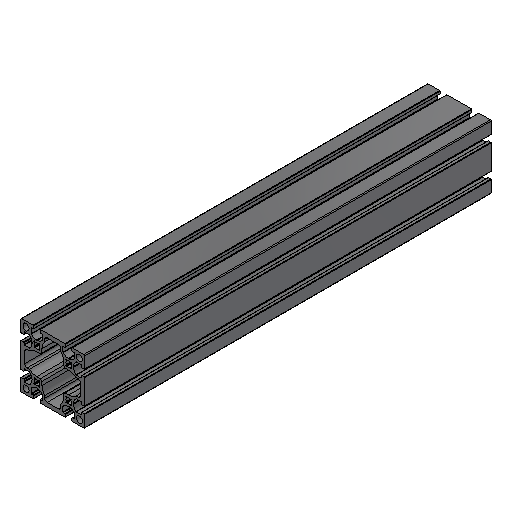
# Autodesk Inventor part: PROFILE
Saved by Autodesk Inventor 2022.5 (Build 265521000, 521)
## iProperties
Created: 2022-06-15
Part Number: PROFILE
Material: AL6061
Document SubType Name: Modeling
Designer: 박성규
Density: 2.71 g/cm^3
Description: 3
MAKER: DY PROFILE
Detail Description: Purchased products
Author: 오동하
Revision Number: A
Title: DP8080-510L
Autodesk Inventor part; units mm, degrees
ref_plane "YZ Plane" through (0, 0, 0) normal (1, 0, 0) x (0, 1, 0)
ref_plane "XZ Plane" through (0, 0, 0) normal (0, 1, 0) x (-1, 0, 0)
ref_plane "XY Plane" through (0, 0, 0) normal (0, 0, 1) x (1, 0, 0)
sketch "스케치3" plane through (0, 0, 0) normal (0, 0, 1) x (1, 0, 0)
  line L0 (20, -40) -> (20, -6.357)
  arc A0 (22.8645, -21.8316) -> (22.906, -22.2062) centre (23.1172, -21.9932) ccw
  circle A1 centre (33.5, -33.5) radius 4
  line L1 (-20, -40) -> (-20, -6.0705)
  arc A2 (22.8645, -21.8316) -> (22.8645, -18.1684) centre (20, -20) ccw
  circle A3 centre (-33.5, -33.5) radius 4
  line L2 (0, -45.1572) -> (0, 0)
  arc A4 (40, 15.3564) -> (39.5, 15.8564) centre (39.5, 15.3564) ccw
  line L3 (39.5, 15.8564) -> (36.5, 15.8564)
  arc A5 (36.5, 15.8564) -> (36, 15.3564) centre (36.5, 15.3564) ccw
  line L4 (36, 15.3564) -> (36, 13.3524)
  arc A6 (35.5, 12.8524) -> (36, 13.3524) centre (35.5, 13.3524) ccw
  line L5 (35.5, 12.8524) -> (29.4329, 12.8524)
  arc A7 (29.0959, 12.9831) -> (29.4329, 12.8524) centre (29.4329, 13.3524) ccw
  arc A8 (26.0139, 19.4861) -> (29.0959, 12.9831) centre (35.5, 20) ccw
  line L6 (26.0139, 19.4861) -> (25.5, 20)
  line L7 (25.5, 20) -> (26.0139, 20.5139)
  arc A9 (29.0959, 27.0169) -> (26.0139, 20.5139) centre (35.5, 20) ccw
  arc A10 (29.4329, 27.1476) -> (29.0959, 27.0169) centre (29.4329, 26.6476) ccw
  line L8 (29.4329, 27.1476) -> (35.5, 27.1476)
  arc A11 (36, 26.6476) -> (35.5, 27.1476) centre (35.5, 26.6476) ccw
  line L9 (36, 26.6476) -> (36, 24.6436)
  arc A12 (36, 24.6436) -> (36.5, 24.1436) centre (36.5, 24.6436) ccw
  line L10 (36.5, 24.1436) -> (39.5, 24.1436)
  arc A13 (39.5, 24.1436) -> (40, 24.6436) centre (39.5, 24.6436) ccw
  line L11 (40, 24.6436) -> (40, 38)
  line L12 (40, 38) -> (40, 39)
  arc A14 (40, 39) -> (39, 40) centre (39, 39) ccw
  line L13 (39, 40) -> (38, 40)
  line L14 (38, 40) -> (24.6436, 40)
  arc A15 (24.6436, 40) -> (24.1436, 39.5) centre (24.6436, 39.5) ccw
  line L15 (24.1436, 39.5) -> (24.1436, 36.5)
  arc A16 (24.1436, 36.5) -> (24.6436, 36) centre (24.6436, 36.5) ccw
  line L16 (24.6436, 36) -> (26.6476, 36)
  arc A17 (27.1476, 35.5) -> (26.6476, 36) centre (26.6476, 35.5) ccw
  line L17 (27.1476, 35.5) -> (27.1476, 29.4329)
  arc A18 (27.0169, 29.0959) -> (27.1476, 29.4329) centre (26.6476, 29.4329) ccw
  arc A19 (20.5139, 26.0139) -> (27.0169, 29.0959) centre (20, 35.5) ccw
  line L18 (20.5139, 26.0139) -> (20, 25.5)
  line L19 (20, 25.5) -> (19.4861, 26.0139)
  arc A20 (12.9831, 29.0959) -> (19.4861, 26.0139) centre (20, 35.5) ccw
  arc A21 (12.8524, 29.4329) -> (12.9831, 29.0959) centre (13.3524, 29.4329) ccw
  line L20 (12.8524, 29.4329) -> (12.8524, 35.5)
  arc A22 (13.3524, 36) -> (12.8524, 35.5) centre (13.3524, 35.5) ccw
  line L21 (13.3524, 36) -> (15.3564, 36)
  arc A23 (15.3564, 36) -> (15.8564, 36.5) centre (15.3564, 36.5) ccw
  line L22 (15.8564, 36.5) -> (15.8564, 39.5)
  arc A24 (15.8564, 39.5) -> (15.3564, 40) centre (15.3564, 39.5) ccw
  line L23 (15.3564, 40) -> (0, 40)
  line L24 (0, 40) -> (-15.3564, 40)
  arc A25 (-15.3564, 40) -> (-15.8564, 39.5) centre (-15.3564, 39.5) ccw
  line L25 (-15.8564, 39.5) -> (-15.8564, 36.5)
  arc A26 (-15.8564, 36.5) -> (-15.3564, 36) centre (-15.3564, 36.5) ccw
  line L26 (-15.3564, 36) -> (-13.3524, 36)
  arc A27 (-12.8524, 35.5) -> (-13.3524, 36) centre (-13.3524, 35.5) ccw
  line L27 (-12.8524, 35.5) -> (-12.8524, 29.4329)
  arc A28 (-12.9831, 29.0959) -> (-12.8524, 29.4329) centre (-13.3524, 29.4329) ccw
  arc A29 (-19.4861, 26.0139) -> (-12.9831, 29.0959) centre (-20, 35.5) ccw
  line L28 (-19.4861, 26.0139) -> (-20, 25.5)
  line L29 (-20, 25.5) -> (-20.5139, 26.0139)
  arc A30 (-27.0169, 29.0959) -> (-20.5139, 26.0139) centre (-20, 35.5) ccw
  arc A31 (-27.1476, 29.4329) -> (-27.0169, 29.0959) centre (-26.6476, 29.4329) ccw
  line L30 (-27.1476, 29.4329) -> (-27.1476, 35.5)
  arc A32 (-26.6476, 36) -> (-27.1476, 35.5) centre (-26.6476, 35.5) ccw
  line L31 (-26.6476, 36) -> (-24.6436, 36)
  arc A33 (-24.6436, 36) -> (-24.1436, 36.5) centre (-24.6436, 36.5) ccw
  line L32 (-24.1436, 36.5) -> (-24.1436, 39.5)
  arc A34 (-24.1436, 39.5) -> (-24.6436, 40) centre (-24.6436, 39.5) ccw
  line L33 (-24.6436, 40) -> (-38, 40)
  line L34 (-38, 40) -> (-39, 40)
  arc A35 (-39, 40) -> (-40, 39) centre (-39, 39) ccw
  line L35 (-40, 39) -> (-40, 38)
  line L36 (-40, 38) -> (-40, 24.6436)
  arc A36 (-40, 24.6436) -> (-39.5, 24.1436) centre (-39.5, 24.6436) ccw
  line L37 (-39.5, 24.1436) -> (-36.5, 24.1436)
  arc A37 (-36.5, 24.1436) -> (-36, 24.6436) centre (-36.5, 24.6436) ccw
  line L38 (-36, 24.6436) -> (-36, 26.6476)
  arc A38 (-35.5, 27.1476) -> (-36, 26.6476) centre (-35.5, 26.6476) ccw
  line L39 (-35.5, 27.1476) -> (-29.4329, 27.1476)
  arc A39 (-29.0959, 27.0169) -> (-29.4329, 27.1476) centre (-29.4329, 26.6476) ccw
  arc A40 (-26.0139, 20.5139) -> (-29.0959, 27.0169) centre (-35.5, 20) ccw
  line L40 (-26.0139, 20.5139) -> (-25.5, 20)
  line L41 (-25.5, 20) -> (-26.0139, 19.4861)
  arc A41 (-29.0959, 12.9831) -> (-26.0139, 19.4861) centre (-35.5, 20) ccw
  arc A42 (-29.4329, 12.8524) -> (-29.0959, 12.9831) centre (-29.4329, 13.3524) ccw
  line L42 (-29.4329, 12.8524) -> (-35.5, 12.8524)
  arc A43 (-36, 13.3524) -> (-35.5, 12.8524) centre (-35.5, 13.3524) ccw
  line L43 (-36, 13.3524) -> (-36, 15.3564)
  arc A44 (-36, 15.3564) -> (-36.5, 15.8564) centre (-36.5, 15.3564) ccw
  line L44 (-36.5, 15.8564) -> (-39.5, 15.8564)
  arc A45 (-39.5, 15.8564) -> (-40, 15.3564) centre (-39.5, 15.3564) ccw
  line L45 (-40, 15.3564) -> (-40, 0)
  line L46 (-40, 0) -> (-40, -15.3564)
  arc A46 (-40, -15.3564) -> (-39.5, -15.8564) centre (-39.5, -15.3564) ccw
  line L47 (-39.5, -15.8564) -> (-36.5, -15.8564)
  arc A47 (-36.5, -15.8564) -> (-36, -15.3564) centre (-36.5, -15.3564) ccw
  line L48 (-36, -15.3564) -> (-36, -13.3524)
  arc A48 (-35.5, -12.8524) -> (-36, -13.3524) centre (-35.5, -13.3524) ccw
  line L49 (-35.5, -12.8524) -> (-29.4329, -12.8524)
  arc A49 (-29.0959, -12.9831) -> (-29.4329, -12.8524) centre (-29.4329, -13.3524) ccw
  arc A50 (-26.0139, -19.4861) -> (-29.0959, -12.9831) centre (-35.5, -20) ccw
  line L50 (-26.0139, -19.4861) -> (-25.5, -20)
  line L51 (-25.5, -20) -> (-26.0139, -20.5139)
  arc A51 (-29.0959, -27.0169) -> (-26.0139, -20.5139) centre (-35.5, -20) ccw
  arc A52 (-29.4329, -27.1476) -> (-29.0959, -27.0169) centre (-29.4329, -26.6476) ccw
  line L52 (-29.4329, -27.1476) -> (-35.5, -27.1476)
  arc A53 (-36, -26.6476) -> (-35.5, -27.1476) centre (-35.5, -26.6476) ccw
  line L53 (-36, -26.6476) -> (-36, -24.6436)
  arc A54 (-36, -24.6436) -> (-36.5, -24.1436) centre (-36.5, -24.6436) ccw
  line L54 (-36.5, -24.1436) -> (-39.5, -24.1436)
  arc A55 (-39.5, -24.1436) -> (-40, -24.6436) centre (-39.5, -24.6436) ccw
  line L55 (-40, -24.6436) -> (-40, -38)
  line L56 (-40, -38) -> (-40, -39)
  arc A56 (-40, -39) -> (-39, -40) centre (-39, -39) ccw
  line L57 (-39, -40) -> (-38, -40)
  line L58 (-38, -40) -> (-24.6436, -40)
  arc A57 (-24.6436, -40) -> (-24.1436, -39.5) centre (-24.6436, -39.5) ccw
  line L59 (-24.1436, -39.5) -> (-24.1436, -36.5)
  arc A58 (-24.1436, -36.5) -> (-24.6436, -36) centre (-24.6436, -36.5) ccw
  line L60 (-24.6436, -36) -> (-26.6476, -36)
  arc A59 (-27.1476, -35.5) -> (-26.6476, -36) centre (-26.6476, -35.5) ccw
  line L61 (-27.1476, -35.5) -> (-27.1476, -29.4329)
  arc A60 (-27.0169, -29.0959) -> (-27.1476, -29.4329) centre (-26.6476, -29.4329) ccw
  arc A61 (-20.5139, -26.0139) -> (-27.0169, -29.0959) centre (-20, -35.5) ccw
  line L62 (-20.5139, -26.0139) -> (-20, -25.5)
  line L63 (-20, -25.5) -> (-19.4861, -26.0139)
  arc A62 (-12.9831, -29.0959) -> (-19.4861, -26.0139) centre (-20, -35.5) ccw
  arc A63 (-12.8524, -29.4329) -> (-12.9831, -29.0959) centre (-13.3524, -29.4329) ccw
  line L64 (-12.8524, -29.4329) -> (-12.8524, -35.5)
  arc A64 (-13.3524, -36) -> (-12.8524, -35.5) centre (-13.3524, -35.5) ccw
  line L65 (-13.3524, -36) -> (-15.3564, -36)
  arc A65 (-15.3564, -36) -> (-15.8564, -36.5) centre (-15.3564, -36.5) ccw
  line L66 (-15.8564, -36.5) -> (-15.8564, -39.5)
  arc A66 (-15.8564, -39.5) -> (-15.3564, -40) centre (-15.3564, -39.5) ccw
  line L67 (-15.3564, -40) -> (0, -40)
  line L68 (0, -40) -> (15.3564, -40)
  arc A67 (15.3564, -40) -> (15.8564, -39.5) centre (15.3564, -39.5) ccw
  line L69 (15.8564, -39.5) -> (15.8564, -36.5)
  arc A68 (15.8564, -36.5) -> (15.3564, -36) centre (15.3564, -36.5) ccw
  line L70 (15.3564, -36) -> (13.3524, -36)
  arc A69 (12.8524, -35.5) -> (13.3524, -36) centre (13.3524, -35.5) ccw
  line L71 (12.8524, -35.5) -> (12.8524, -29.4329)
  arc A70 (12.9831, -29.0959) -> (12.8524, -29.4329) centre (13.3524, -29.4329) ccw
  arc A71 (19.4861, -26.0139) -> (12.9831, -29.0959) centre (20, -35.5) ccw
  line L72 (19.4861, -26.0139) -> (20, -25.5)
  line L73 (20, -25.5) -> (20.5139, -26.0139)
  arc A72 (27.0169, -29.0959) -> (20.5139, -26.0139) centre (20, -35.5) ccw
  arc A73 (27.1476, -29.4329) -> (27.0169, -29.0959) centre (26.6476, -29.4329) ccw
  line L74 (27.1476, -29.4329) -> (27.1476, -35.5)
  arc A74 (26.6476, -36) -> (27.1476, -35.5) centre (26.6476, -35.5) ccw
  line L75 (26.6476, -36) -> (24.6436, -36)
  arc A75 (24.6436, -36) -> (24.1436, -36.5) centre (24.6436, -36.5) ccw
  line L76 (24.1436, -36.5) -> (24.1436, -39.5)
  arc A76 (24.1436, -39.5) -> (24.6436, -40) centre (24.6436, -39.5) ccw
  line L77 (24.6436, -40) -> (38, -40)
  line L78 (38, -40) -> (39, -40)
  arc A77 (39, -40) -> (40, -39) centre (39, -39) ccw
  line L79 (40, -39) -> (40, -38)
  line L80 (40, -38) -> (40, -24.6436)
  arc A78 (40, -24.6436) -> (39.5, -24.1436) centre (39.5, -24.6436) ccw
  line L81 (39.5, -24.1436) -> (36.5, -24.1436)
  arc A79 (36.5, -24.1436) -> (36, -24.6436) centre (36.5, -24.6436) ccw
  line L82 (36, -24.6436) -> (36, -26.6476)
  arc A80 (35.5, -27.1476) -> (36, -26.6476) centre (35.5, -26.6476) ccw
  line L83 (35.5, -27.1476) -> (29.4329, -27.1476)
  arc A81 (29.0959, -27.0169) -> (29.4329, -27.1476) centre (29.4329, -26.6476) ccw
  arc A82 (26.0139, -20.5139) -> (29.0959, -27.0169) centre (35.5, -20) ccw
  line L84 (26.0139, -20.5139) -> (25.5, -20)
  line L85 (25.5, -20) -> (26.0139, -19.4861)
  arc A83 (29.0959, -12.9831) -> (26.0139, -19.4861) centre (35.5, -20) ccw
  arc A84 (29.4329, -12.8524) -> (29.0959, -12.9831) centre (29.4329, -13.3524) ccw
  line L86 (29.4329, -12.8524) -> (35.5, -12.8524)
  arc A85 (36, -13.3524) -> (35.5, -12.8524) centre (35.5, -13.3524) ccw
  line L87 (36, -13.3524) -> (36, -15.3564)
  arc A86 (36, -15.3564) -> (36.5, -15.8564) centre (36.5, -15.3564) ccw
  line L88 (36.5, -15.8564) -> (39.5, -15.8564)
  arc A87 (39.5, -15.8564) -> (40, -15.3564) centre (39.5, -15.3564) ccw
  line L89 (40, -15.3564) -> (40, 0)
  line L90 (40, 0) -> (40, 15.3564)
  arc A88 (22.906, -17.7938) -> (22.8645, -18.1684) centre (23.1172, -18.0068) ccw
  line L91 (22.906, -17.7938) -> (23.6045, -17.1009)
  arc A89 (35, 7) -> (32, 10) centre (32, 7) ccw
  line L92 (32, 10) -> (29.0692, 10)
  arc A90 (29.0692, 10) -> (20, 13.5) centre (20, 0) ccw
  line L93 (20, 13.5) -> (15.4691, 13.5)
  line L94 (15.4691, 13.5) -> (13.5, 15.4691)
  line L95 (13.5, 15.4691) -> (13.5, 20)
  arc A91 (13.5, 20) -> (10, 29.0692) centre (0, 20) ccw
  line L96 (10, 29.0692) -> (10, 32)
  arc A92 (10, 32) -> (7, 35) centre (7, 32) ccw
  line L97 (7, 35) -> (0, 35)
  line L98 (0, 35) -> (-7, 35)
  arc A93 (-7, 35) -> (-10, 32) centre (-7, 32) ccw
  line L99 (-10, 32) -> (-10, 29.0692)
  arc A94 (-10, 29.0692) -> (-13.5, 20) centre (0, 20) ccw
  line L100 (-13.5, 20) -> (-13.5, 15.4691)
  line L101 (-13.5, 15.4691) -> (-15.4691, 13.5)
  line L102 (-15.4691, 13.5) -> (-20, 13.5)
  arc A95 (-20, 13.5) -> (-29.0692, 10) centre (-20, 0) ccw
  line L103 (-29.0692, 10) -> (-32, 10)
  arc A96 (-32, 10) -> (-35, 7) centre (-32, 7) ccw
  line L104 (-35, 7) -> (-35, 0)
  line L105 (-35, 0) -> (-35, -7)
  arc A97 (-35, -7) -> (-32, -10) centre (-32, -7) ccw
  line L106 (-32, -10) -> (-29.0692, -10)
  arc A98 (-29.0692, -10) -> (-20, -13.5) centre (-20, 0) ccw
  line L107 (-20, -13.5) -> (-15.4691, -13.5)
  line L108 (-15.4691, -13.5) -> (-13.5, -15.4691)
  line L109 (-13.5, -15.4691) -> (-13.5, -20)
  arc A99 (-13.5, -20) -> (-10, -29.0692) centre (0, -20) ccw
  line L110 (-10, -29.0692) -> (-10, -32)
  arc A100 (-10, -32) -> (-7, -35) centre (-7, -32) ccw
  line L111 (-7, -35) -> (0, -35)
  line L112 (0, -35) -> (7, -35)
  arc A101 (7, -35) -> (10, -32) centre (7, -32) ccw
  line L113 (10, -32) -> (10, -29.0692)
  arc A102 (10, -29.0692) -> (13.5, -20) centre (0, -20) ccw
  line L114 (13.5, -20) -> (13.5, -15.4691)
  line L115 (13.5, -15.4691) -> (15.4691, -13.5)
  line L116 (15.4691, -13.5) -> (20, -13.5)
  arc A103 (20, -13.5) -> (29.0692, -10) centre (20, 0) ccw
  line L117 (29.0692, -10) -> (32, -10)
  arc A104 (32, -10) -> (35, -7) centre (32, -7) ccw
  line L118 (35, -7) -> (35, 0)
  line L119 (35, 0) -> (35, 7)
  circle A105 centre (-33.5, 33.5) radius 4
  line L120 (0, 45.1572) -> (0, 0)
  line L121 (0, 0) -> (-45.8762, 0)
  line L122 (-20, 40) -> (-20, 5.3913)
  arc A106 (-17.094, 22.2062) -> (-17.1355, 21.8316) centre (-16.8828, 21.9932) ccw
  line L123 (-17.094, 22.2062) -> (-16.3955, 22.8991)
  arc A107 (-16.3955, 22.8991) -> (-16.3946, 23.3243) centre (-16.6067, 23.1121) ccw
  line L124 (-16.3946, 23.3243) -> (-16.6757, 23.6054)
  arc A108 (-16.6757, 23.6054) -> (-17.1009, 23.6045) centre (-16.8879, 23.3933) ccw
  line L125 (-17.1009, 23.6045) -> (-17.7938, 22.906)
  arc A109 (-18.1684, 22.8645) -> (-17.7938, 22.906) centre (-18.0068, 23.1172) ccw
  arc A110 (-18.1684, 22.8645) -> (-21.8316, 22.8645) centre (-20, 20) ccw
  arc A111 (-22.2062, 22.906) -> (-21.8316, 22.8645) centre (-21.9932, 23.1172) ccw
  line L126 (-22.2062, 22.906) -> (-22.8991, 23.6045)
  arc A112 (-22.8991, 23.6045) -> (-23.3243, 23.6054) centre (-23.1121, 23.3933) ccw
  line L127 (-23.3243, 23.6054) -> (-23.6054, 23.3243)
  arc A113 (-23.6054, 23.3243) -> (-23.6045, 22.8991) centre (-23.3933, 23.1121) ccw
  line L128 (-23.6045, 22.8991) -> (-22.906, 22.2062)
  arc A114 (-22.8645, 21.8316) -> (-22.906, 22.2062) centre (-23.1172, 21.9932) ccw
  arc A115 (-22.8645, 21.8316) -> (-22.8645, 18.1684) centre (-20, 20) ccw
  arc A116 (-22.906, 17.7938) -> (-22.8645, 18.1684) centre (-23.1172, 18.0068) ccw
  line L129 (-22.906, 17.7938) -> (-23.6045, 17.1009)
  arc A117 (-23.6045, 17.1009) -> (-23.6054, 16.6757) centre (-23.3933, 16.8879) ccw
  line L130 (-23.6054, 16.6757) -> (-23.3243, 16.3946)
  arc A118 (-23.3243, 16.3946) -> (-22.8991, 16.3955) centre (-23.1121, 16.6067) ccw
  line L131 (-22.8991, 16.3955) -> (-22.2062, 17.094)
  arc A119 (-21.8316, 17.1355) -> (-22.2062, 17.094) centre (-21.9932, 16.8828) ccw
  arc A120 (-21.8316, 17.1355) -> (-18.1684, 17.1355) centre (-20, 20) ccw
  arc A121 (-17.7938, 17.094) -> (-18.1684, 17.1355) centre (-18.0068, 16.8828) ccw
  line L132 (-17.7938, 17.094) -> (-17.1009, 16.3955)
  arc A122 (-17.1009, 16.3955) -> (-16.6757, 16.3946) centre (-16.8879, 16.6067) ccw
  line L133 (-16.6757, 16.3946) -> (-16.3946, 16.6757)
  arc A123 (-16.3946, 16.6757) -> (-16.3955, 17.1009) centre (-16.6067, 16.8879) ccw
  line L134 (-16.3955, 17.1009) -> (-17.094, 17.7938)
  arc A124 (-17.1355, 18.1684) -> (-17.094, 17.7938) centre (-16.8828, 18.0068) ccw
  arc A125 (-17.1355, 18.1684) -> (-17.1355, 21.8316) centre (-20, 20) ccw
  line L135 (-17.094, -17.7938) -> (-16.3955, -17.1009)
  arc A126 (-16.3955, -17.1009) -> (-16.3946, -16.6757) centre (-16.6067, -16.8879) ccw
  line L136 (-16.3946, -16.6757) -> (-16.6757, -16.3946)
  arc A127 (-16.6757, -16.3946) -> (-17.1009, -16.3955) centre (-16.8879, -16.6067) ccw
  line L137 (-17.1009, -16.3955) -> (-17.7938, -17.094)
  arc A128 (-18.1684, -17.1355) -> (-17.7938, -17.094) centre (-18.0068, -16.8828) ccw
  arc A129 (-18.1684, -17.1355) -> (-21.8316, -17.1355) centre (-20, -20) ccw
  arc A130 (-22.2062, -17.094) -> (-21.8316, -17.1355) centre (-21.9932, -16.8828) ccw
  line L138 (-22.2062, -17.094) -> (-22.8991, -16.3955)
  arc A131 (-22.8991, -16.3955) -> (-23.3243, -16.3946) centre (-23.1121, -16.6067) ccw
  line L139 (-23.3243, -16.3946) -> (-23.6054, -16.6757)
  arc A132 (-23.6054, -16.6757) -> (-23.6045, -17.1009) centre (-23.3933, -16.8879) ccw
  line L140 (-23.6045, -17.1009) -> (-22.906, -17.7938)
  arc A133 (-22.8645, -18.1684) -> (-22.906, -17.7938) centre (-23.1172, -18.0068) ccw
  arc A134 (-22.8645, -18.1684) -> (-22.8645, -21.8316) centre (-20, -20) ccw
  arc A135 (-22.906, -22.2062) -> (-22.8645, -21.8316) centre (-23.1172, -21.9932) ccw
  line L141 (-22.906, -22.2062) -> (-23.6045, -22.8991)
  arc A136 (-23.6045, -22.8991) -> (-23.6054, -23.3243) centre (-23.3933, -23.1121) ccw
  line L142 (-23.6054, -23.3243) -> (-23.3243, -23.6054)
  arc A137 (-23.3243, -23.6054) -> (-22.8991, -23.6045) centre (-23.1121, -23.3933) ccw
  line L143 (-22.8991, -23.6045) -> (-22.2062, -22.906)
  arc A138 (-21.8316, -22.8645) -> (-22.2062, -22.906) centre (-21.9932, -23.1172) ccw
  arc A139 (-21.8316, -22.8645) -> (-18.1684, -22.8645) centre (-20, -20) ccw
  arc A140 (-17.7938, -22.906) -> (-18.1684, -22.8645) centre (-18.0068, -23.1172) ccw
  line L144 (-17.7938, -22.906) -> (-17.1009, -23.6045)
  arc A141 (-17.1009, -23.6045) -> (-16.6757, -23.6054) centre (-16.8879, -23.3933) ccw
  line L145 (-16.6757, -23.6054) -> (-16.3946, -23.3243)
  arc A142 (-16.3946, -23.3243) -> (-16.3955, -22.8991) centre (-16.6067, -23.1121) ccw
  line L146 (-16.3955, -22.8991) -> (-17.094, -22.2062)
  arc A143 (-17.1355, -21.8316) -> (-17.094, -22.2062) centre (-16.8828, -21.9932) ccw
  arc A144 (-17.1355, -21.8316) -> (-17.1355, -18.1684) centre (-20, -20) ccw
  arc A145 (-17.094, -17.7938) -> (-17.1355, -18.1684) centre (-16.8828, -18.0068) ccw
  line L147 (20, 40) -> (20, 5.6778)
  circle A146 centre (33.5, 33.5) radius 4
  arc A147 (22.906, 22.2062) -> (22.8645, 21.8316) centre (23.1172, 21.9932) ccw
  line L148 (22.906, 22.2062) -> (23.6045, 22.8991)
  arc A148 (23.6045, 22.8991) -> (23.6054, 23.3243) centre (23.3933, 23.1121) ccw
  line L149 (23.6054, 23.3243) -> (23.3243, 23.6054)
  arc A149 (23.3243, 23.6054) -> (22.8991, 23.6045) centre (23.1121, 23.3933) ccw
  line L150 (22.8991, 23.6045) -> (22.2062, 22.906)
  arc A150 (21.8316, 22.8645) -> (22.2062, 22.906) centre (21.9932, 23.1172) ccw
  arc A151 (21.8316, 22.8645) -> (18.1684, 22.8645) centre (20, 20) ccw
  arc A152 (17.7938, 22.906) -> (18.1684, 22.8645) centre (18.0068, 23.1172) ccw
  line L151 (17.7938, 22.906) -> (17.1009, 23.6045)
  arc A153 (17.1009, 23.6045) -> (16.6757, 23.6054) centre (16.8879, 23.3933) ccw
  line L152 (16.6757, 23.6054) -> (16.3946, 23.3243)
  arc A154 (16.3946, 23.3243) -> (16.3955, 22.8991) centre (16.6067, 23.1121) ccw
  line L153 (16.3955, 22.8991) -> (17.094, 22.2062)
  arc A155 (17.1355, 21.8316) -> (17.094, 22.2062) centre (16.8828, 21.9932) ccw
  arc A156 (17.1355, 21.8316) -> (17.1355, 18.1684) centre (20, 20) ccw
  arc A157 (17.094, 17.7938) -> (17.1355, 18.1684) centre (16.8828, 18.0068) ccw
  line L154 (17.094, 17.7938) -> (16.3955, 17.1009)
  arc A158 (16.3955, 17.1009) -> (16.3946, 16.6757) centre (16.6067, 16.8879) ccw
  line L155 (16.3946, 16.6757) -> (16.6757, 16.3946)
  arc A159 (16.6757, 16.3946) -> (17.1009, 16.3955) centre (16.8879, 16.6067) ccw
  line L156 (17.1009, 16.3955) -> (17.7938, 17.094)
  arc A160 (18.1684, 17.1355) -> (17.7938, 17.094) centre (18.0068, 16.8828) ccw
  arc A161 (18.1684, 17.1355) -> (21.8316, 17.1355) centre (20, 20) ccw
  arc A162 (22.2062, 17.094) -> (21.8316, 17.1355) centre (21.9932, 16.8828) ccw
  line L157 (22.2062, 17.094) -> (22.8991, 16.3955)
  arc A163 (22.8991, 16.3955) -> (23.3243, 16.3946) centre (23.1121, 16.6067) ccw
  line L158 (23.3243, 16.3946) -> (23.6054, 16.6757)
  arc A164 (23.6054, 16.6757) -> (23.6045, 17.1009) centre (23.3933, 16.8879) ccw
  line L159 (23.6045, 17.1009) -> (22.906, 17.7938)
  arc A165 (22.8645, 18.1684) -> (22.906, 17.7938) centre (23.1172, 18.0068) ccw
  arc A166 (22.8645, 18.1684) -> (22.8645, 21.8316) centre (20, 20) ccw
  arc A167 (23.6045, -17.1009) -> (23.6054, -16.6757) centre (23.3933, -16.8879) ccw
  line L160 (23.6054, -16.6757) -> (23.3243, -16.3946)
  arc A168 (23.3243, -16.3946) -> (22.8991, -16.3955) centre (23.1121, -16.6067) ccw
  line L161 (22.8991, -16.3955) -> (22.2062, -17.094)
  arc A169 (21.8316, -17.1355) -> (22.2062, -17.094) centre (21.9932, -16.8828) ccw
  arc A170 (21.8316, -17.1355) -> (18.1684, -17.1355) centre (20, -20) ccw
  arc A171 (17.7938, -17.094) -> (18.1684, -17.1355) centre (18.0068, -16.8828) ccw
  line L162 (17.7938, -17.094) -> (17.1009, -16.3955)
  arc A172 (17.1009, -16.3955) -> (16.6757, -16.3946) centre (16.8879, -16.6067) ccw
  line L163 (16.6757, -16.3946) -> (16.3946, -16.6757)
  arc A173 (16.3946, -16.6757) -> (16.3955, -17.1009) centre (16.6067, -16.8879) ccw
  line L164 (16.3955, -17.1009) -> (17.094, -17.7938)
  arc A174 (17.1355, -18.1684) -> (17.094, -17.7938) centre (16.8828, -18.0068) ccw
  arc A175 (17.1355, -18.1684) -> (17.1355, -21.8316) centre (20, -20) ccw
  arc A176 (17.094, -22.2062) -> (17.1355, -21.8316) centre (16.8828, -21.9932) ccw
  line L165 (17.094, -22.2062) -> (16.3955, -22.8991)
  arc A177 (16.3955, -22.8991) -> (16.3946, -23.3243) centre (16.6067, -23.1121) ccw
  line L166 (16.3946, -23.3243) -> (16.6757, -23.6054)
  arc A178 (16.6757, -23.6054) -> (17.1009, -23.6045) centre (16.8879, -23.3933) ccw
  line L167 (17.1009, -23.6045) -> (17.7938, -22.906)
  arc A179 (18.1684, -22.8645) -> (17.7938, -22.906) centre (18.0068, -23.1172) ccw
  arc A180 (18.1684, -22.8645) -> (21.8316, -22.8645) centre (20, -20) ccw
  arc A181 (22.2062, -22.906) -> (21.8316, -22.8645) centre (21.9932, -23.1172) ccw
  line L168 (22.2062, -22.906) -> (22.8991, -23.6045)
  arc A182 (22.8991, -23.6045) -> (23.3243, -23.6054) centre (23.1121, -23.3933) ccw
  line L169 (23.3243, -23.6054) -> (23.6054, -23.3243)
  arc A183 (23.6054, -23.3243) -> (23.6045, -22.8991) centre (23.3933, -23.1121) ccw
  line L170 (23.6045, -22.8991) -> (22.906, -22.2062)
  line L171 (33.5, -35.5) -> (33.5, -38.5)
  line L172 (-33.5, -35.5) -> (-33.5, -38.5)
  line L173 (41.0297, 20) -> (4.21, 20)
  line L174 (41.0297, -20) -> (5.357, -20)
  line L175 (-33.5, -31.5) -> (-33.5, -28.5)
  line L176 (-31.5, 33.5) -> (-28.5, 33.5)
  line L177 (-33.5, 31.5) -> (-33.5, 28.5)
  line L178 (-35.5, 33.5) -> (-38.5, 33.5)
  line L179 (-33.5, 35.5) -> (-33.5, 38.5)
  line L180 (-41.0297, 20) -> (-4.393, 20)
  line L181 (-15.6747, 24.3253) -> (-24.3253, 15.6747)
  line L182 (-24.3253, 24.3253) -> (-15.6747, 15.6747)
  line L183 (-33.5, 32.5) -> (-33.5, 34.5)
  line L184 (-32.5, 33.5) -> (-34.5, 33.5)
  line L185 (-41.0297, -20) -> (-5.8268, -20)
  line L186 (-35.5, -33.5) -> (-38.5, -33.5)
  line L187 (-15.6747, -24.3253) -> (-24.3253, -15.6747)
  line L188 (-24.3253, -24.3253) -> (-15.6747, -15.6747)
  line L189 (-31.5, -33.5) -> (-28.5, -33.5)
  line L190 (35.5, 33.5) -> (38.5, 33.5)
  line L191 (-32.5, -33.5) -> (-34.5, -33.5)
  line L192 (-33.5, -32.5) -> (-33.5, -34.5)
  line L193 (33.5, 32.5) -> (33.5, 34.5)
  line L194 (24.3253, 24.3253) -> (15.6747, 15.6747)
  line L195 (15.6747, 24.3253) -> (24.3253, 15.6747)
  line L196 (31.5, 33.5) -> (28.5, 33.5)
  line L197 (32.5, 33.5) -> (34.5, 33.5)
  line L198 (33.5, 31.5) -> (33.5, 28.5)
  line L199 (33.5, 35.5) -> (33.5, 38.5)
  line L200 (24.3253, -24.3253) -> (15.6747, -15.6747)
  line L201 (15.6747, -24.3253) -> (24.3253, -15.6747)
  line L202 (31.5, -33.5) -> (28.5, -33.5)
  line L203 (33.5, -32.5) -> (33.5, -34.5)
  line L204 (33.5, -31.5) -> (33.5, -28.5)
  line L205 (32.5, -33.5) -> (34.5, -33.5)
  line L206 (35.5, -33.5) -> (38.5, -33.5)
  point P0 (0, 0)
  constraints: 414 end point, 360 point on circle, 184 centre point, 22 point on line
extrude "돌출1" add sketch "스케치3" along normal mid plane 510 contours L72 A71 A70 L71 A69 L70 A68 L69 A67 L68 L2 L112 A101 L113 A102 L174 A175 A176 L165 A177 L166 A178 L167 A179 A180 L0 | L0 A180 A181 L168 A182 L169 A183 L170 A0 A2 L174 L84 A82 A81 L83 A80 L82 A79 L81 A78 L80 L79 A77 L78 L77 A76 L76 A75 L75 A74 L74 A73 A72 L73 | A170 A171 L162 A172 L163 A173 L164 A174 A175 L174 L114 L115 L116 L0 | L0 A103 L117 A104 L118 L119 A89 L92 A90 L147 A161 A162 L157 A163 L158 A164 L159 A165 A166 L173 L6 A8 A7 L5 A6 L4 A5 L3 A4 L90 L89 A87 L88 A86 L87 A85 L86 A84 A83 L85 L174 A2 A88 L91 A167 L160 A168 L161 A169 A170 | L2 L67 A66 L66 A65 L65 A64 L64 A63 A62 L63 L1 A139 A140 L144 A141 L145 A142 L146 A143 A144 L185 A99 L110 A100 L111 | L120 L23 A24 L22 A23 L21 A22 L20 A21 A20 L19 L147 A151 A152 L151 A153 L152 A154 L153 A155 A156 L173 A91 L96 A92 L97 | L98 A93 L99 A94 L180 A125 A106 L123 A107 L124 A108 L125 A109 A110 L122 L28 A29 A28 L27 A27 L26 A26 L25 A25 L24 L120 | L121 L45 A45 L44 A44 L43 A43 L42 A42 A41 L41 L180 A115 A116 L129 A117 L130 A118 L131 A119 A120 L122 A95 L103 A96 L104 | L105 A97 L106 A98 L1 A129 A130 L138 A131 L139 A132 L140 A133 A134 L185 L50 A50 A49 L49 A48 L48 A47 L47 A46 L46 L121 | L93 L94 L95 L173 A156 A157 L154 A158 L155 A159 L156 A160 A161 L147 | L185 A144 A145 L135 A126 L136 A127 L137 A128 A129 L1 L107 L108 L109 | L100 L101 L102 L122 A120 A121 L132 A122 L133 A123 L134 A124 A125 L180 | L147 L18 A19 A18 L17 A17 L16 A16 L15 A15 L14 L13 A14 L12 L11 A13 L10 A12 L9 A11 L8 A10 A9 L7 L173 A166 A147 L148 A148 L149 A149 L150 A150 A151 | L1 L62 A61 A60 L61 A59 L60 A58 L59 A57 L58 L57 A56 L56 L55 A55 L54 A54 L53 A53 L52 A52 A51 L51 L185 A134 A135 L141 A136 L142 A137 L143 A138 A139 | A110 A111 L126 A112 L127 A113 L128 A114 A115 L180 L40 A40 A39 L39 A38 L38 A37 L37 A36 L36 L35 A35 L34 L33 A34 L32 A33 L31 A32 L30 A31 A30 L29 L122
